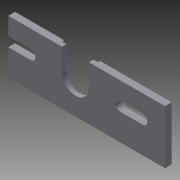
# Autodesk Inventor part: JHeadMount
Saved by Autodesk Inventor 2014 SP1 (Build 180222100, 222)
## iProperties
Created: 2014-01-05
Part Number: JHeadMount
Material: Aluminum 6061
Document SubType Name: Modeling
Designer: Jack
Density: 2.71 g/cm^3
Appearance: Aluminum - Flat
Author: Jack
Autodesk Inventor part; units mm, degrees
ref_plane "YZ Plane" through (0, 0, 0) normal (1, 0, 0) x (0, 1, 0)
ref_plane "XZ Plane" through (0, 0, 0) normal (0, 1, 0) x (-1, 0, 0)
ref_plane "XY Plane" through (0, 0, 0) normal (0, 0, 1) x (1, 0, 0)
sketch "Sketch1" plane through (0, 0, 0) normal (0, 1, 0) x (-1, 0, 0)
  line L0 (0, 0) -> (70, 0)
  line L1 (70, 0) -> (70, 24)
  line L2 (70, 24) -> (0, 24)
  line L3 (0, 24) -> (0, 0)
  dimension "d0" = 70
  dimension "d1" = 24
  constraints: 8 end point, 2 perpendicular, 1 horizontal, 1 parallel
  measures "d0" distance of L0.start L0.end
  measures "d1" distance of L0.end L1.end
extrude "Extrusion1" add sketch "Sketch1" along normal blind 3
sketch "Sketch2" plane through (0, 3, 0) normal (0, 1, 0) x (1, 0, 0)
  line L0 (-70, 0) -> (-70, -24) projected
  line L1 (-70, -24) -> (0, -24) projected
  arc A0 (-32, -14) -> (-48, -14) centre (-40, -14) ccw
  line L2 (-32, -14) -> (-32, -24)
  line L3 (-48, -14) -> (-48, -24)
  dimension "d5" = 16
  dimension "d6" = 10
  dimension "d8" = 30
  constraints: 4 end point, 2 perpendicular, 2 point on circle, 2 point on line, 2 tangent, 1 centre point
  measures "d5" diameter of A0
  measures "d6" distance from line of L1 A0.centre
  measures "d8" distance from line of L0 A0.centre
extrude "Extrusion2" cut sketch "Sketch2" against normal blind 1
sketch "Sketch3" plane through (0, 2, 0) normal (0, 1, 0) x (1, 0, 0)
  arc A0 (-32, -14) -> (-48, -14) centre (-40, -14) ccw projected
  line L0 (-32, -24) -> (-48, -24) projected
  arc A1 (-34, -14) -> (-46, -14) centre (-40, -14) ccw
  line L1 (-46, -14) -> (-46, -24)
  line L2 (-34, -14) -> (-34, -24)
  point P0 (0, 0)
  dimension "d11" = 12
  constraints: 4 end point, 2 perpendicular, 2 point on circle, 2 point on line, 2 tangent, 1 centre point, 1 coincident
  measures "d11" diameter of A1
extrude "Extrusion3" cut sketch "Sketch3" against normal blind 2
sketch "Sketch4" plane through (0, 3, 0) normal (0, 1, 0) x (1, 0, 0)
  line L0 (-32, -24) -> (0, -24) projected
  line L1 (0, -24) -> (0, 0) projected
  line L2 (-70, 0) -> (-70, -24) projected
  arc A0 (-32, -14) -> (-48, -14) centre (-40, -14) ccw projected
  line L3 (-70, -14) -> (-60, -14) construction
  line L4 (-70, -16.15) -> (-60, -16.15)
  line L5 (-60, -11.85) -> (-70, -11.85)
  arc A1 (-70, -11.85) -> (-70, -16.15) centre (-70, -14) ccw
  arc A2 (-60, -16.15) -> (-60, -11.85) centre (-60, -14) ccw
  line L6 (-20, -14) -> (-10, -14) construction
  line L7 (-20, -16.15) -> (-10, -16.15)
  line L8 (-10, -11.85) -> (-20, -11.85)
  arc A3 (-20, -11.85) -> (-20, -16.15) centre (-20, -14) ccw
  arc A4 (-10, -16.15) -> (-10, -11.85) centre (-10, -14) ccw
  point P0 (-65, -14)
  point P1 (-15, -14)
  dimension "d14" = 5
  dimension "d15" = 4.3
  dimension "d16" = 5
  dimension "d17" = 5
  dimension "d18" = 4.3
  dimension "d19" = 15
  constraints: 16 end point, 8 point on circle, 8 tangent, 4 centre point, 4 parallel, 2 horizontal alignment, 2 midpoint
  measures "d14" distance of point (-65, -14) L3.end
  measures "d15" diameter of A2
  measures "d16" distance from line of L2 point (-65, -14)
  measures "d17" distance of point (-15, -14) L6.end
  measures "d18" diameter of A4
  measures "d19" distance from line of L1 point (-15, -14)
extrude "Extrusion4" cut sketch "Sketch4" against normal blind 3
body "Solid1"
